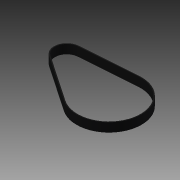
# Autodesk Inventor part: belt
Saved by Autodesk Inventor 2014 SP1 (Build 180222100, 222)
## iProperties
Created: 2014-05-23
Part Number: belt
Material: Generic
Document SubType Name: Modeling
Designer: brent
Density: 1 g/cm^3
Appearance: Default
d0: 1.000 ul
d1: 2.506 in
d4: 0.940 in
d8: 2.458 in
d11: 0.354 in
d12: 0.00 deg
d0_1: 1.000 ul
d2: 0.866 in
d3: 0.169 in
d5: 0.866 in
d6: 2.598 in
d7: 2.458 in
d13: 4.000 ul
d17: 2.454 in
d18: 1.904 in
motor_hole_distance: 22.000 mm
center_to_center_distance: 2.458 in
mount_thickness: 0.500 in
motor_diameter: 2.205 in
mount_motor_thickness: 0.125 in
board_mount_clearance: 0.605 in
motor_tension_increment: 0.075 in
motor_tension_holeoffset: 0.500 in
largepulley_diameter: 63.660 mm
smallpulley_diameter: 23.870 mm
d15: 360.00 deg
Author: brent
Autodesk Inventor part; units mm, degrees
ref_plane "YZ Plane" through (0, 0, 0) normal (1, 0, 0) x (0, 1, 0)
ref_plane "XZ Plane" through (0, 0, 0) normal (0, 1, 0) x (-1, 0, 0)
ref_plane "XY Plane" through (0, 0, 0) normal (0, 0, 1) x (1, 0, 0)
derived "mountsketch_alt.ipt"
sketch "Sketch1" plane through (0, 0, 0) normal (0, 1, 0) x (-1, 0, 0)
  arc A0 (-20.0089, 38.3403) -> (-35.6242, -19.9447) centre (-37.6152, 11.823) ccw
  arc A1 (23.4303, -16.2436) -> (29.2855, 5.611) centre (22.6838, -4.332) ccw
  line L0 (-19.1548, 38.9712) -> (29.5905, 5.8251)
  line L1 (29.2855, 5.611) -> (-20.0089, 38.3403)
  line L2 (23.4303, -16.2436) -> (-35.6242, -19.9447)
  arc A2 (23.5874, -16.5816) -> (29.5905, 5.8251) centre (22.6838, -4.332) ccw
  line L3 (-35.2, -20.9181) -> (23.5874, -16.5816)
  arc A3 (-19.1548, 38.9712) -> (-35.2, -20.9181) centre (-37.6152, 11.823) ccw
  point P0 (0, 0)
  dimension "d1" = 63.66
  dimension "d4" = 23.87
  dimension "d8" = 62.4256
  constraints: 8 end point, 8 point on circle, 8 tangent, 4 centre point, 2 coincident
  measures "d1" diameter of A0
  measures "d4" diameter of A1
  measures "d8" distance of A1.centre A0.centre
extrude "Extrusion1" add sketch "Sketch1" along normal blind 9
equation "\"d1\" = largepulley_diameter"
equation "\"d4\" = smallpulley_diameter"
equation "\"d8\" = center_to_center_distance"
equation "\"largepulley_diameter\" = 63.66"
equation "\"smallpulley_diameter\" = 23.87"
equation "\"center_to_center_distance\" = 62.42558"
body "Solid1"
